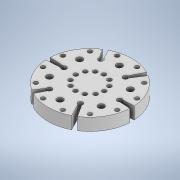
# Autodesk Inventor part: Part10
Saved by Autodesk Inventor 2021 (Build 250183000, 183)
## iProperties
Created: 2022-04-24
Part Number: Part10
Material: Generic
Document SubType Name: Modeling
Designer: hp
Density: 1 g/cm^3
Appearance: Default
Author: hp
Autodesk Inventor part; units mm, degrees
ref_plane "YZ Plane" through (0, 0, 0) normal (1, 0, 0) x (0, 1, 0)
ref_plane "XZ Plane" through (0, 0, 0) normal (0, 1, 0) x (-1, 0, 0)
ref_plane "XY Plane" through (0, 0, 0) normal (0, 0, 1) x (1, 0, 0)
sketch "Sketch1" plane through (0, 0, 0) normal (0, 1, 0) x (-1, 0, 0)
  arc A0 (18.5177, -28.5148) -> (33.9534, -1.7794) centre (0, 0) ccw
  circle A1 centre (29.9437, -8.0234) radius 1.75
  circle A2 centre (21.9203, -21.9203) radius 1.75
  circle A3 centre (20.659, -12.215) radius 2.5
  circle A4 centre (9.8159, -5.9548) radius 1.75
  arc A5 (13.9011, -21.4058) -> (11, -19.0526) centre (12, -20.7846) ccw
  arc A6 (9.75, 0) -> (13.25, 0) centre (11.5, 0) ccw
  arc A7 (6.625, -11.4748) -> (4.875, -8.4437) centre (5.75, -9.9593) ccw
  arc A8 (19, 0) -> (22.6111, -1.185) centre (21, 0) ccw
  line L0 (33.9681, -1.7802) -> (22.6111, -1.185)
  line L1 (18.5177, -28.5148) -> (13.9011, -21.4058)
  arc A9 (33.9534, 1.7794) -> (18.5177, 28.5148) centre (0, 0) ccw
  circle A10 centre (29.9437, 8.0234) radius 1.75
  circle A11 centre (21.9203, 21.9203) radius 1.75
  circle A12 centre (20.659, 12.215) radius 2.5
  circle A13 centre (9.8159, 5.9548) radius 1.75
  arc A14 (11, 19.0526) -> (13.9011, 21.4058) centre (12, 20.7846) ccw
  arc A15 (13.25, 0) -> (9.75, 0) centre (11.5, 0) ccw
  arc A16 (4.875, 8.4437) -> (6.625, 11.4748) centre (5.75, 9.9593) ccw
  arc A17 (22.6111, 1.185) -> (19, 0) centre (21, 0) ccw
  line L2 (33.9681, 1.7802) -> (22.6111, 1.185)
  line L3 (18.5177, 28.5148) -> (13.9011, 21.4058)
  arc A18 (-15.4357, -30.2942) -> (15.4357, -30.2942) centre (0, 0) ccw
  circle A19 centre (-8.0234, -29.9437) radius 1.75
  circle A20 centre (8.0234, -29.9437) radius 1.75
  circle A21 centre (0.2491, -23.9987) radius 2.5
  circle A22 centre (0.2491, -11.4783) radius 1.75
  arc A23 (11, -19.0526) -> (11.5874, -22.7416) centre (12, -20.7846) ccw
  arc A24 (-6.625, -11.4748) -> (-4.875, -8.4437) centre (-5.75, -9.9593) ccw
  arc A25 (4.875, -8.4437) -> (6.625, -11.4748) centre (5.75, -9.9593) ccw
  arc A26 (-10.2793, -20.1743) -> (-9.5, -16.4545) centre (-10.5, -18.1865) ccw
  line L4 (-15.4424, -30.3073) -> (-10.2793, -20.1743)
  line L5 (15.4357, -30.2942) -> (11.5874, -22.7416)
  arc A27 (-18.5177, 28.5148) -> (-33.9534, 1.7794) centre (0, 0) ccw
  circle A28 centre (-21.9203, 21.9203) radius 1.75
  circle A29 centre (-29.9437, 8.0234) radius 1.75
  circle A30 centre (-20.908, 11.7837) radius 2.5
  circle A31 centre (-10.065, 5.5234) radius 1.75
  arc A32 (-22, 0) -> (-25.4885, 1.3358) centre (-24, 0) ccw
  arc A33 (-6.625, 11.4748) -> (-4.875, 8.4437) centre (-5.75, 9.9593) ccw
  arc A34 (-9.75, 0) -> (-13.25, 0) centre (-11.5, 0) ccw
  line L6 (-13.25, 0) -> (-22, 0)
  arc A35 (-12.3318, 18.9893) -> (-9.5, 16.4545) centre (-10.5, 18.1865) ccw
  line L7 (-18.5257, 28.5271) -> (-12.3318, 18.9893)
  line L8 (-33.9534, 1.7794) -> (-25.4885, 1.3358)
  arc A36 (6.625, 11.4748) -> (4.875, 8.4437) centre (5.75, 9.9593) ccw
  arc A37 (11.5874, 22.7416) -> (11, 19.0526) centre (12, 20.7846) ccw
  circle A38 centre (8.0234, 29.9437) radius 1.75
  line L9 (15.4357, 30.2942) -> (11.5874, 22.7416)
  circle A39 centre (0.2491, 11.4783) radius 1.75
  arc A40 (-4.875, 8.4437) -> (-6.625, 11.4748) centre (-5.75, 9.9593) ccw
  arc A41 (-9.5, 16.4545) -> (-10.2793, 20.1743) centre (-10.5, 18.1865) ccw
  circle A42 centre (0.2491, 23.9987) radius 2.5
  arc A43 (15.4357, 30.2942) -> (-15.4357, 30.2942) centre (0, 0) ccw
  circle A44 centre (-8.0234, 29.9437) radius 1.75
  line L10 (-15.4424, 30.3073) -> (-10.2793, 20.1743)
  arc A45 (-4.875, -8.4437) -> (-6.625, -11.4748) centre (-5.75, -9.9593) ccw
  circle A46 centre (-10.065, -5.5234) radius 1.75
  arc A47 (-13.25, 0) -> (-9.75, 0) centre (-11.5, 0) ccw
  arc A48 (-9.5, -16.4545) -> (-12.3318, -18.9893) centre (-10.5, -18.1865) ccw
  arc A49 (-25.4885, -1.3358) -> (-22, 0) centre (-24, 0) ccw
  circle A50 centre (-20.908, -11.7837) radius 2.5
  circle A51 centre (-29.9437, -8.0234) radius 1.75
  arc A52 (-33.9534, -1.7794) -> (-18.5177, -28.5148) centre (0, 0) ccw
  line L11 (-33.9534, -1.7794) -> (-25.4885, -1.3358)
  circle A53 centre (-21.9203, -21.9203) radius 1.75
  line L12 (-18.5257, -28.5271) -> (-12.3318, -18.9893)
  constraints: 60 point on circle, 54 centre point, 26 end point, 8 coincident, 7 point on line
extrude "Extrusion1" add sketch "Sketch1" along normal blind 10
body "Solid1"
